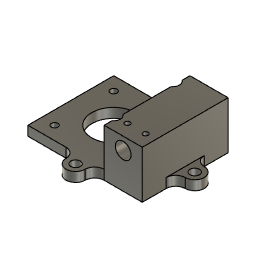
Y-Motor (Autodesk Fusion 360 design; units mm, degrees)
Autodesk Fusion 360 part; units mm, degrees
note: some values were not read from the file. Set by a fixed rule: which sketch regions a step uses.
sketch "Skizze1" plane through (0, 0, 0) normal (0, 0, 1) x (1, 0, 0)
  line L0 (0, 0) -> (60, 0)
  line L1 (60, 0) -> (60, 45)
  line L2 (60, 45) -> (0, 45)
  line L3 (0, 45) -> (0, 0)
  dimension "d1" = 60
  dimension "d2" = 45
  constraint horizontal L0
  constraint vertical L1
  constraint horizontal L2
  constraint vertical L3
  constraint coincident L0.start L3.end
  measures "d1" distance of L0.start L0.end
  measures "d2" distance of L0.start L2.end
extrude "Extrusion1" add sketch "Skizze1" along normal blind 5
sketch "Skizze2" plane through (0, 0, 5) normal (0, 0, 1) x (-1, 0, 0)
  line L0 (0, -45) -> (0, 0)
  line L1 (0, 0) -> (-60, 0)
  line L2 (-60, 0) -> (-60, -45)
  line L3 (-60, -45) -> (0, -45)
  line L4 (0, 0) -> (-45, 0)
  line L5 (-45, 0) -> (-45, -45)
  line L6 (-45, -45) -> (0, -45)
  line L7 (0, -45) -> (0, 0)
  line L8 (-22.5, -45) -> (-22.5, 0)
  line L9 (0, -22.5) -> (-45, -22.5)
  circle A0 centre (-22.5, -22.5) radius 11.5
  line L10 (-22.5, -22.5) -> (-7, -22.5)
  line L11 (-7, -22.5) -> (-7, -38)
  line L12 (-7, -38) -> (-22.5, -38)
  line L13 (-22.5, -38) -> (-22.5, -22.5)
  line L14 (-22.5, -38) -> (-38, -38)
  line L15 (-38, -38) -> (-38, -7)
  line L16 (-7, -22.5) -> (-7, -7)
  line L17 (-38, -7) -> (-7, -7)
  circle A1 centre (-7, -38) radius 1.75
  circle A2 centre (-38, -38) radius 1.75
  circle A3 centre (-38, -7) radius 1.75
  circle A4 centre (-7, -7) radius 1.75
  dimension "d7" = 23
  dimension "d8" = 15.5
  dimension "d9" = 15.5
  dimension "d10" = 31
  dimension "d11" = 3.5
  constraint horizontal L4
  constraint vertical L5
  constraint horizontal L6
  constraint vertical L7
  constraint coincident L0.end L1.start
  constraint midpoint L6 L8.start
  constraint midpoint L4 L8.end
  constraint midpoint L7 L9.start
  constraint midpoint L5 L9.end
  constraint equal L2 L7
  constraint equal L2 L4
  constraint midpoint L8 A0.centre
  constraint horizontal L10
  constraint vertical L11
  constraint horizontal L12
  constraint vertical L13
  constraint coincident A0.centre L10.start
  constraint perpendicular L8 L14
  constraint perpendicular L12 L15
  constraint equal L12 L14
  constraint perpendicular L10 L16
  constraint equal L11 L16
  constraint coincident L11.end L12.start
  constraint coincident L14.end L15.start
  constraint coincident L15.end L17.start
  constraint coincident L16.end L17.end
  constraint equal A1 A2
  constraint equal A2 A3
  constraint equal A3 A4
  measures "d7" diameter of A0
  measures "d8" distance of A0.centre L10.end
  measures "d9" distance of A0.centre L12.end
  measures "d10" distance of L14.end L15.end
  measures "d11" diameter of A1
extrude "Extrusion2" cut sketch "Skizze2" against normal blind 5 contours L8 L9 A0 L10 L13 | L8 L9 A0 L10 | L11 L12 A1 | L11 L12 A1 | L16 L17 A4 | L16 L17 A4 | L8 L9 A0 L13 | L14 L15 A2 | L14 L15 A2 | L8 L9 A0 | L15 L17 A3 | L15 L17 A3
sketch "Skizze3" plane through (0, 0, 5) normal (0, 0, 1) x (-1, 0, 0)
  circle A0 centre (-22.5, -22.5) radius 11.5
  circle A1 centre (-38, -38) radius 1.75
  circle A2 centre (-38, -7) radius 1.75
  circle A3 centre (-7, -38) radius 1.75
  circle A4 centre (-7, -7) radius 1.75
  line L0 (0, -45) -> (0, 0)
  line L1 (0, 0) -> (-60, 0)
  line L2 (-60, 0) -> (-60, -45)
  line L3 (-60, -45) -> (0, -45)
  line L4 (-60, 0) -> (-40, 0)
  line L5 (-40, -45) -> (-60, -45)
  line L6 (-60, -45) -> (-60, 0)
  line L7 (-40, -40.8723) -> (-40, -45)
  arc A5 (-40, -35.1277) -> (-40, -40.8723) centre (-38, -38) ccw
  line L8 (-40, 0) -> (-40, -4.1277)
  line L9 (-40, -9.8723) -> (-40, -35.1277)
  arc A6 (-40, -4.1277) -> (-40, -9.8723) centre (-38, -7) ccw
  dimension "d14" = 20
  dimension "d15" = 7
  dimension "d16" = 7
  constraint horizontal L4
  constraint vertical L8
  constraint horizontal L5
  constraint vertical L6
  constraint coincident L1.end L2.start
  constraint concentric A1 A5
  constraint concentric A2 A6
  constraint collinear L7 L8
  constraint collinear L8 L9
  measures "d14" distance of L1.end L4.end
  measures "d15" diameter of A5
  measures "d16" diameter of A6
extrude "Extrusion3" add sketch "Skizze3" along normal blind 20 contours L1 L2 L3 L4 L5 L6 L7 A5 L8 L9 A6
sketch "Skizze4" plane through (0, 0, 0) normal (0, 0, -1) x (1, 0, 0)
  circle A0 centre (22.5, -22.5) radius 11.5
  circle A1 centre (38, -38) radius 1.75
  circle A2 centre (38, -7) radius 1.75
  circle A3 centre (7, -38) radius 1.75
  circle A4 centre (7, -7) radius 1.75
  line L0 (0, 0) -> (0, -45)
  line L1 (0, -45) -> (60, -45)
  line L2 (60, -45) -> (60, 0)
  line L3 (60, 0) -> (0, 0)
  line L4 (60, -22.5) -> (70, -22.5)
  line L5 (30, -45) -> (30, -55)
  line L6 (30, -50) -> (40, -50)
  line L7 (40, -50) -> (30, -50)
  line L8 (30, -50) -> (20, -50)
  line L9 (65, -22.5) -> (65, -12.5)
  line L10 (65, -22.5) -> (65, -32.5)
  circle A5 centre (65, -22.5) radius 5
  circle A6 centre (30, -50) radius 5
  circle A7 centre (20, -50) radius 5
  circle A8 centre (40, -50) radius 5
  circle A9 centre (65, -12.5) radius 5
  circle A10 centre (65, -32.5) radius 5
  circle A11 centre (30, -50) radius 2.5
  circle A12 centre (65, -22.5) radius 2.5
  line L11 (30, 0) -> (30, 10)
  line L12 (30, 5) -> (40, 5)
  line L13 (30, 5) -> (20, 5)
  circle A13 centre (30, 5) radius 5
  circle A14 centre (20, 5) radius 5
  circle A15 centre (40, 5) radius 5
  circle A16 centre (30, 5) radius 2.5
  dimension "d19" = 10
  dimension "d20" = 10
  dimension "d21" = 10
  dimension "d22" = 10
  dimension "d27" = 5
  dimension "d28" = 5
  dimension "d35" = 10
  dimension "d36" = 10
  dimension "d37" = 5
  constraint midpoint L2 L4.start
  constraint perpendicular L2 L4
  constraint midpoint L1 L5.start
  constraint perpendicular L1 L5
  constraint midpoint L5 L6.start
  constraint perpendicular L5 L6
  constraint perpendicular L5 L8
  constraint equal L5 L8
  constraint equal L5 L6
  constraint midpoint L4 L9.start
  constraint perpendicular L4 L9
  constraint perpendicular L4 L10
  constraint equal L4 L9
  constraint equal L4 L10
  constraint coincident L9.start L10.start
  constraint coincident L6.start L7.end
  constraint coincident L8.end A7.centre
  constraint coincident L6.end L7.start
  constraint coincident L9.end A9.centre
  constraint coincident L10.end A10.centre
  constraint equal A6 A7
  constraint equal A6 A8
  constraint equal A5 A10
  constraint equal A5 A9
  constraint concentric A5 A12
  constraint midpoint L3 L11.start
  constraint perpendicular L3 L11
  constraint midpoint L11 L12.start
  constraint perpendicular L11 L12
  constraint perpendicular L11 L13
  constraint equal L11 L13
  constraint equal L11 L12
  constraint coincident L12.start L13.start
  constraint coincident L13.end A14.centre
  constraint coincident L12.end A15.centre
  constraint equal A13 A14
  constraint equal A13 A15
  measures "d19" distance of L4.start L4.end
  measures "d20" distance of L5.start L5.end
  measures "d21" diameter of A5
  measures "d22" diameter of A6
  measures "d27" diameter of A11
  measures "d28" diameter of A12
  measures "d35" distance of L11.start L11.end
  measures "d36" diameter of A13
  measures "d37" diameter of A16
extrude "Extrusion4" add sketch "Skizze4" against normal blind 5 contours L3 A13 A14 | L3 A13 A15 | L11 L13 A13 A16 | L11 L12 A13 A16 | L11 L13 A13 A16 | L11 L12 A13 A16 | L2 A5 A9 | L2 A5 A10 | L4 L9 A5 A12 | L4 L10 A5 A12 | L4 L9 A5 A12 | L4 L10 A5 A12
sketch "Skizze5" plane through (0, 45, 0) normal (0, 1, 0) x (-1, 0, 0)
  line L0 (-40, 5) -> (-40, 25)
  line L1 (-40, 25) -> (-60, 25)
  line L2 (-60, 25) -> (-60, 0)
  line L3 (-60, 0) -> (0, 0)
  line L4 (-30, 0) -> (-30, 18.5)
  circle A0 centre (-30, 18.5) radius 4.15
  line L5 (0, 0) -> (0, 5)
  line L6 (0, 5) -> (-40, 5)
  dimension "d31" = 18.5
  dimension "d32" = 8.3
  constraint midpoint L3 L4.start
  constraint perpendicular L3 L4
  constraint coincident L4.end A0.centre
  measures "d31" distance of L4.start L4.end
  measures "d32" diameter of A0
extrude "Extrusion5" cut sketch "Skizze5" against normal blind 6 contours A0
sketch "Skizze6" plane through (0, 0, 0) normal (0, -1, 0) x (1, 0, 0)
  line L0 (40, 5) -> (40, 0)
  line L1 (40, 0) -> (60, 0)
  line L2 (60, 0) -> (60, 25)
  line L3 (60, 25) -> (40, 25)
  line L4 (40, 25) -> (40, 5)
  line L5 (50, 0) -> (50, 18.5)
  circle A0 centre (50, 18.5) radius 4.15
  dimension "d38" = 18.5
  dimension "d39" = 8.3
  constraint midpoint L1 L5.start
  constraint perpendicular L1 L5
  constraint coincident L5.end A0.centre
  measures "d38" distance of L5.start L5.end
  measures "d39" diameter of A0
extrude "Extrusion6" cut sketch "Skizze6" against normal blind 6 contours A0
sketch "Skizze8" plane through (0, 0, 25) normal (0, 0, 1) x (-1, 0, 0)
  line L0 (-40, -4.1277) -> (-40, 0)
  line L1 (-40, 0) -> (-60, 0)
  line L2 (-60, 0) -> (-60, -45)
  line L3 (-60, -45) -> (-40, -45)
  line L4 (-40, -45) -> (-40, -40.8723)
  arc A0 (-40, -35.1277) -> (-40, -40.8723) centre (-38, -38) ccw
  line L5 (-40, -35.1277) -> (-40, -9.8723)
  arc A1 (-40, -4.1277) -> (-40, -9.8723) centre (-38, -7) ccw
  line L6 (-50, 0) -> (-50, -7)
  line L7 (-50, -7) -> (-45.25, -7)
  line L8 (-50, -7) -> (-54.75, -7)
  circle A2 centre (-45.25, -7) radius 1.35
  circle A3 centre (-54.75, -7) radius 1.35
  dimension "d42" = 7
  dimension "d43" = 4.75
  dimension "d44" = 2.7
  dimension "d45" = 2.7
  constraint midpoint L1 L6.start
  constraint perpendicular L1 L6
  constraint perpendicular L6 L7
  constraint perpendicular L6 L8
  constraint equal L7 L8
  constraint coincident L7.end A2.centre
  constraint coincident L8.end A3.centre
  measures "d42" distance of L6.start L6.end
  measures "d43" distance of L6.end L7.end
  measures "d44" diameter of A2
  measures "d45" diameter of A3
extrude "Extrusion7" cut sketch "Skizze8" against normal blind 5 contours A2 | A3
